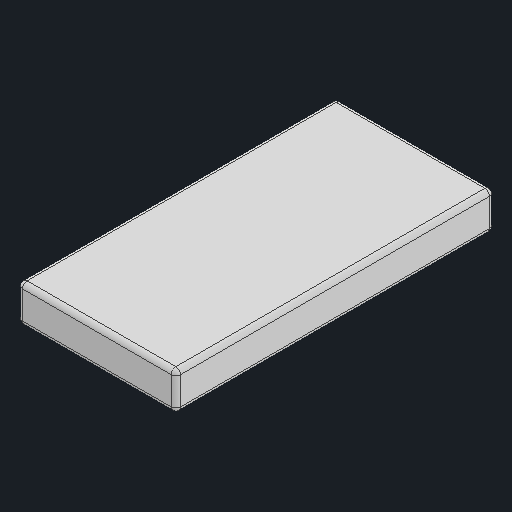
# Autodesk Inventor part: Battery_Large
Saved by Autodesk Inventor 2026.2 (Build 302298000, 298)
## iProperties
Created: 2026-02-04
Part Number: Battery_Large
Material: Generic
Document SubType Name: Modeling
Designer: vckot
Density: 1 g/cm^3
Appearance: Default
Author: vckot
Autodesk Inventor part; units mm, degrees
ref_plane "YZ Plane" through (0, 0, 0) normal (1, 0, 0) x (0, 1, 0)
ref_plane "XZ Plane" through (0, 0, 0) normal (0, 1, 0) x (-1, 0, 0)
ref_plane "XY Plane" through (0, 0, 0) normal (0, 0, 1) x (1, 0, 0)
sketch "Sketch1" plane through (0, 0, 0) normal (0, 1, 0) x (-1, 0, 0)
  line L0 (34, 68.5) -> (-34, 68.5)
  line L1 (-34, 68.5) -> (-34, -68.5)
  line L2 (-34, -68.5) -> (34, -68.5)
  line L3 (34, -68.5) -> (34, 68.5)
  line L4 (34, 68.5) -> (-34, -68.5) construction
  line L5 (-34, 68.5) -> (34, -68.5) construction
  point P0 (0, 0)
  dimension "d0" = 68
  dimension "d1" = 137
  constraints: 12 end point, 2 midpoint, 2 parallel, 1 horizontal, 1 perpendicular
  measures "d0" distance of L2.end L1.end
  measures "d1" distance of L1.end L0.end
extrude "Extrusion1" add sketch "Sketch1" along normal blind 16
fillet "Fillet1" radius 2 3 edges at (0, 16, 68.5) (34, 16, 0) (34, 8, 68.5)
fillet "Fillet1" radius 2 12 edges at (-34, 8, 68.5) (34, 8, 68.5) (0, 0, 68.5) (0, 16, 68.5) (-34, 8, -68.5) (-34, 0, 0) (-34, 16, 0) (34, 8, -68.5) (0, 0, -68.5) (0, 16, -68.5) (34, 0, 0) (34, 16, 0)
body "Solid1"
